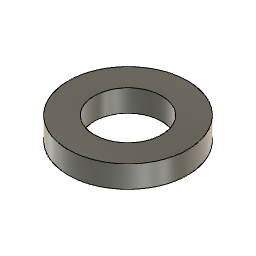
timing_pulley_spacer (Autodesk Fusion 360 design; units mm, degrees)
Autodesk Fusion 360 part; units mm, degrees
sketch "Sketch1" plane through (0, 0, 0) normal (0, 0, 1) x (1, 0, 0) in component "support"
  circle A0 centre (0, 0) radius 2.6
  circle A1 centre (0, 0) radius 4.6
  dimension "d1" = 5.2
  dimension "d2" = 2
  constraint coincident A0.centre A1.centre
  measures "d1" diameter of A0
extrude "Extrude1" add sketch "Sketch1" along normal blind 1.7 in component "support"
component "support" placed x (1, 0, 0) y (0, 1, 0) z (0, 0, 1) at (0, 0, 0)
